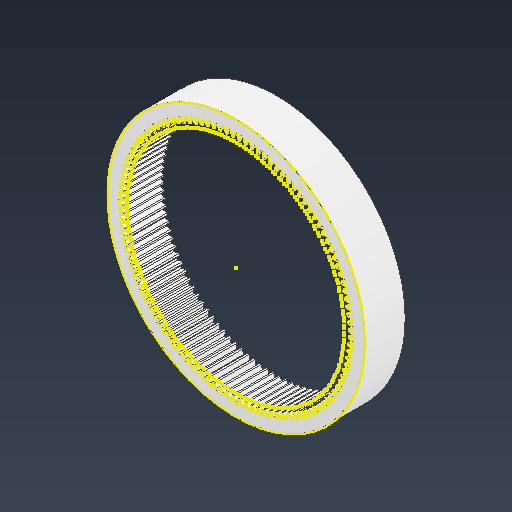
# Autodesk Inventor part: 平歯車2
Saved by Autodesk Inventor 2021 (Build 250183000, 183)
## iProperties
CustomPartVersion: 1
Created: 2021-08-20
Part Number: 平歯車2
Material: Steel
Document SubType Name: Modeling
Designer: yuta0
Categories: <?xml version="1.0" encoding="UTF-16"?> <MemberInstance><Categories><FamilyTemplate><FamilyTemplateParameter ValueType="xs:double" Id="1" ObjectReferenceKey="da_z" ObjectType="kUserParameterObject"/><FamilyTemplateParameter ValueType="xs:double" Id="2" ObjectReferenceKey="da_b" ObjectType="kUserParameterObject"/><FamilyTemplateParameter ValueType="xs:double" Id="3" ObjectReferenceKey="da_beta" ObjectType="kUserParameterObject"/><FamilyTemplateParameter ValueType="xs:double" Id="4" ObjectReferenceKey="da_da" ObjectType="kUserParameterObject"/><FamilyTemplateParameter ValueType="xs:double" Id="5" ObjectReferenceKey="da_aw" ObjectType="kUserParameterObject"/><FamilyTemplateParameter ValueType="xs:string" Id="6" ObjectReferenceKey="EAIAABAAAACIAQAAAAAAAIAAAAAAAAAA" ObjectType="83910656" SubObjectId="SurfaceGeometry"/></FamilyTemplate><ParamToTemplateMap><ParamToTemplate CategoryParameter="//CategoryParameter[@InternalName='046C89C9-8512-4d59-83FE-43B91F4F132A']" TemplateParameter="1"/><ParamToTemplate CategoryParameter="//CategoryParameter[@InternalName='2552DF32-E462-4b46-AEBF-C6C7768E72AC']" TemplateParameter="2"/><ParamToTemplate CategoryParameter="//CategoryParameter[@InternalName='C9EE641D-15FC-4fae-A226-E94C4372FDD7']" TemplateParameter="3"/><ParamToTemplate><ParamToTemplate CategoryParameter="//CategoryParameter[@InternalName='00B6519A-459B-49c7-AD84-2E56D39A5744']" ConstantValue="0.135415"/></ParamToTemplate><ParamToTemplate><ParamToTemplate CategoryParameter="//CategoryParameter[@InternalName='04B31F0E-C7A6-4894-AA32-9629BEFACF47']" ConstantValue="1.000000"/></ParamToTemplate><ParamToTemplate><ParamToTemplate CategoryParameter="//CategoryParameter[@InternalName='43CBEC2E-7847-49e7-A936-2F7889FCB2D9']" ConstantValue="0.250000"/></ParamToTemplate><ParamToTemplate><ParamToTemplate CategoryParameter="//CategoryParameter[@InternalName='B1EFC894-105D-4ebd-86BF-FA20ED196853']" ConstantValue="0.350000"/></ParamToTemplate><ParamToTemplate><ParamToTemplate CategoryParameter="//CategoryParameter[@InternalName='51175063-3D10-4879-93E8-6246FE8B403D']" ConstantValue="2060000000.000000"/></ParamToTemplate><ParamToTemplate><ParamToTemplate CategoryParameter="//CategoryParameter[@InternalName='A3A52E27-4454-46a9-B0BD-C932399B70AF']" ConstantValue="0.300000"/></ParamToTemplate><ParamToTemplate><ParamToTemplate CategoryParameter="//CategoryParameter[@InternalName='91B76062-C214-41d9-B1B9-14D2AB99603D']" ConstantValue="0.100000"/></ParamToTemplate><ParamToTemplate><ParamToTemplate CategoryParameter="//CategoryParameter[@InternalName='374E806E-8B8A-4dda-A9AA-1039D6500AD2']" ConstantValue="10.000000"/></ParamToTemplate><ParamToTemplate><ParamToTemplate CategoryParameter="//CategoryParameter[@InternalName='2D373A89-B862-43d6-8D0B-0CBF12AB9F6C']" ConstantValue="0.349066"/></ParamToTemplate><ParamToTemplate CategoryParameter="//CategoryParameter[@InternalName='37777632-D6A2-4fac-9D53-DB8ACD95C989']" TemplateParameter="4"/><ParamToTemplate CategoryParameter="//CategoryParameter[@InternalName='FD1017F1-B727-4f7e-9707-0F86F1FF9423']" TemplateParameter="5"/><ParamToTemplate><ParamToTemplate CategoryParameter="//CategoryParameter[@InternalName='9E1B4470-B2D3-4ff1-B813-535BB4CDF51A']" ConstantValue="3520000.000000"/></ParamToTemplate><ParamToTemplate><ParamToTemplate CategoryParameter="//CategoryParameter[@InternalName='F8452263-BFF6-458c-9FB1-07C4B99E95CD']" ConstantValue="11400000.000000"/></ParamToTemplate><ParamToTemplate><ParamToTemplate CategoryParameter="//CategoryParameter[@InternalName='3E3BB259-FD49-497f-8171-6EBC954A3479']" ConstantValue="2.000000"/></ParamToTemplate><ParamToTemplate CategoryParameter="//CategoryParameter[@InternalName='27C3BAF2-7550-4e4b-AE2C-0DB134B7D9B7']" TemplateParameter="6"/></ParamToTemplateMap><Category DisplayName="Gear" InternalName="DC85795E-93AB-48d5-8EEE-5A27447B64BD" Mnemonic="Gear"><CategoryParameter DisplayName="z" InternalName="046C89C9-8512-4d59-83FE-43B91F4F132A" Mnemonic="z"/><CategoryParameter DisplayName="b" InternalName="2552DF32-E462-4b46-AEBF-C6C7768E72AC" Mnemonic="b"/><CategoryParameter DisplayName="||b|" InternalName="C9EE641D-15FC-4fae-A226-E94C4372FDD7" Mnemonic="beta"/><CategoryParameter DisplayName="x" InternalName="00B6519A-459B-49c7-AD84-2E56D39A5744" Mnemonic="x"/><CategoryParameter DisplayName="a*" InternalName="04B31F0E-C7A6-4894-AA32-9629BEFACF47" Mnemonic="a"/><CategoryParameter DisplayName="c*" InternalName="43CBEC2E-7847-49e7-A936-2F7889FCB2D9" Mnemonic="c"/><CategoryParameter DisplayName="r|.f|*" InternalName="B1EFC894-105D-4ebd-86BF-FA20ED196853" Mnemonic="rf"/><CategoryParameter DisplayName="E" InternalName="51175063-3D10-4879-93E8-6246FE8B403D" Mnemonic="E"/><CategoryParameter DisplayName="||m|" InternalName="A3A52E27-4454-46a9-B0BD-C932399B70AF" Mnemonic="mi"/><Category DisplayName="SpurGear" InternalName="26C5A22E-A91E-4dfd-A3B3-23CCAFAE1764" Mnemonic="SpurGear"><CategoryParameter DisplayName="m" InternalName="91B76062-C214-41d9-B1B9-14D2AB99603D" Mnemonic="m"/><CategoryParameter DisplayName="P" InternalName="374E806E-8B8A-4dda-A9AA-1039D6500AD2" Mnemonic="PP"/><CategoryParameter DisplayName="||a|" InternalName="2D373A89-B862-43d6-8D0B-0CBF12AB9F6C" Mnemonic="alpha"/><CategoryParameter DisplayName="d|.a|" InternalName="37777632-D6A2-4fac-9D53-DB8ACD95C989" Mnemonic="da"/><CategoryParameter DisplayName="a|.w|" InternalName="FD1017F1-B727-4f7e-9707-0F86F1FF9423" Mnemonic="aw"/><CategoryParameter DisplayName="||s||.Flim|" InternalName="9E1B4470-B2D3-4ff1-B813-535BB4CDF51A" Mnemonic="sFlim"/><CategoryParameter DisplayName="||s||.Hlim|" InternalName="F8452263-BFF6-458c-9FB1-07C4B99E95CD" Mnemonic="sHlim"/><CategoryParameter DisplayName="種類" InternalName="3E3BB259-FD49-497f-8171-6EBC954A3479" Mnemonic="type"/><Category DisplayName="InternalSpurGear" InternalName="7CF704F6-14A9-42f8-93CE-E71DF57C2B55" Mnemonic="InternalSpurGear"><CategoryParameter DisplayName="PitchDiameter" InternalName="27C3BAF2-7550-4e4b-AE2C-0DB134B7D9B7" Mnemonic="IDS_PITCHDIAM"/></Category></Category></Category></Categories></MemberInstance>
Density: 1 g/cm^3
Appearance: 積雪
Author: yuta0
Autodesk Inventor part; units mm, degrees
sketch "Sketch1" plane through (0, 0, 0) normal (0, 0, 1) x (1, 0, 0)
  circle A0 centre (0, 0) radius 63.124
  dimension "d0" = 126.2479
  constraints: 1 centre point
  measures "d0" diameter of A0
extrude "Extrusion1" add sketch "Sketch1" along normal blind 20
ref_plane "Work Plane2" through (0, 0, 10) normal (0, 0, 1) x (1, 0, 0)
sketch "Sketch2" plane through (0, 0, 0) normal (0, 0, -1) x (-1, 0, 0)
  circle A0 centre (0, 0) radius 63.124 projected
  circle A1 centre (0, 0) radius 56
  dimension "d3" = 112
  constraints: 1 centre point, 1 coincident
  measures "d3" diameter of A1
surface extrude "ピッチ円直径" sketch "Sketch2" against normal through all shown no curves A1
ref_plane "Work Plane8" through (0, 0, 0) normal (0.9996066, 0.0280463, 0) x (0, 0, 1)
ref_plane "Work Plane9" through (0, 0, 0) normal (1, 0, 0) x (0, 1, 0)
spur gear teeth "平歯車" teeth 112 pitch diameter 112 tip diameter 110.2708 root diameter 114.7708 face width 20 start plane through (0, 0, 0) normal (0, 0, -1) x (-1, 0, 0)
sketch "スケッチ3" plane through (0, 0, 20) normal (0, 0, 1) x (1, 0, 0)
  arc A0 (3.6193, -57.2712) -> (4.2488, -54.9715) centre (-9.8202, -52.3566) ccw projected
  arc A1 (2.8158, -57.3163) -> (3.6193, -57.2712) centre (0, 0) ccw projected
  arc A2 (1.9328, -55.1015) -> (2.8158, -57.3163) centre (15.6206, -50.9279) ccw projected
  arc A3 (1.1598, -55.1232) -> (1.9328, -55.1015) centre (0, 0) ccw projected
  arc A4 (0.4024, -57.384) -> (1.1598, -55.1232) centre (-12.7405, -51.7236) ccw projected
  arc A5 (-0.4024, -57.384) -> (0.4024, -57.384) centre (0, 0) ccw projected
  arc A6 (-1.1598, -55.1232) -> (-0.4024, -57.384) centre (12.7405, -51.7236) ccw projected
  arc A7 (-1.9328, -55.1015) -> (-1.1598, -55.1232) centre (0, 0) ccw projected
  arc A8 (-2.8158, -57.3163) -> (-1.9328, -55.1015) centre (-15.6206, -50.9279) ccw projected
  arc A9 (-3.6193, -57.2712) -> (-2.8158, -57.3163) centre (0, 0) ccw projected
  arc A10 (-4.2488, -54.9715) -> (-3.6193, -57.2712) centre (9.8202, -52.3566) ccw projected
  arc A11 (-5.0193, -54.9065) -> (-4.2488, -54.9715) centre (0, 0) ccw projected
  arc A12 (-6.0251, -57.0682) -> (-5.0193, -54.9065) centre (-18.4516, -49.9719) ccw projected
  arc A13 (-6.8249, -56.9781) -> (-6.0251, -57.0682) centre (0, 0) ccw projected
  arc A14 (-7.3244, -54.6468) -> (-6.8249, -56.9781) centre (6.8691, -52.8248) ccw projected
  arc A15 (-8.09, -54.5387) -> (-7.3244, -54.6468) centre (0, 0) ccw projected
  arc A16 (-9.2155, -56.6406) -> (-8.09, -54.5387) centre (-21.2245, -48.8587) ccw projected
  arc A17 (-10.0089, -56.5058) -> (-9.2155, -56.6406) centre (0, 0) ccw projected
  arc A18 (-10.3769, -54.1501) -> (-10.0089, -56.5058) centre (3.8964, -53.1269) ccw projected
  arc A19 (-11.1353, -53.9992) -> (-10.3769, -54.1501) centre (0, 0) ccw projected
  arc A20 (-12.3768, -56.0348) -> (-11.1353, -53.9992) centre (-23.9306, -47.5918) ccw projected
  arc A21 (-13.1615, -55.8557) -> (-12.3768, -56.0348) centre (0, 0) ccw projected
  arc A22 (-13.3968, -53.4831) -> (-13.1615, -55.8557) centre (0.9114, -53.2618) ccw projected
  arc A23 (-14.1456, -53.2899) -> (-13.3968, -53.4831) centre (0, 0) ccw projected
  arc A24 (-15.4992, -55.2527) -> (-14.1456, -53.2899) centre (-26.5615, -46.1751) ccw projected
  arc A25 (-16.2726, -55.0299) -> (-15.4992, -55.2527) centre (0, 0) ccw projected
  arc A26 (-16.3746, -52.6478) -> (-16.2726, -55.0299) centre (-2.0764, -53.2291) ccw projected
  arc A27 (-17.1113, -52.4129) -> (-16.3746, -52.6478) centre (0, 0) ccw projected
  arc A28 (-18.5729, -54.2967) -> (-17.1113, -52.4129) centre (-29.1087, -44.6131) ccw projected
  arc A29 (-19.3326, -54.0309) -> (-18.5729, -54.2967) centre (0, 0) ccw projected
  arc A30 (-19.3008, -51.6468) -> (-19.3326, -54.0309) centre (-5.0577, -53.0289) ccw projected
  arc A31 (-20.0232, -51.3711) -> (-19.3008, -51.6468) centre (0, 0) ccw projected
  arc A32 (-21.5881, -53.1699) -> (-20.0232, -51.3711) centre (-31.5644, -42.9108) ccw projected
  arc A33 (-22.3317, -52.8619) -> (-21.5881, -53.1699) centre (0, 0) ccw projected
  arc A34 (-22.1663, -50.4834) -> (-22.3317, -52.8619) centre (-8.0231, -52.6619) ccw projected
  arc A35 (-22.8721, -50.1675) -> (-22.1663, -50.4834) centre (0, 0) ccw projected
  arc A36 (-24.5354, -51.8758) -> (-22.8721, -50.1675) centre (-33.9208, -41.0735) ccw projected
  arc A37 (-25.2605, -51.5266) -> (-24.5354, -51.8758) centre (0, 0) ccw projected
  arc A38 (-24.962, -49.1611) -> (-25.2605, -51.5266) centre (-10.9633, -52.1292) ccw projected
  arc A39 (-25.649, -48.8062) -> (-24.962, -49.1611) centre (0, 0) ccw projected
  arc A40 (-27.4055, -50.4185) -> (-25.649, -48.8062) centre (-36.1704, -39.1069) ccw projected
  arc A41 (-28.1099, -50.0292) -> (-27.4055, -50.4185) centre (0, 0) ccw projected
  arc A42 (-27.6792, -47.6841) -> (-28.1099, -50.0292) centre (-13.8689, -51.4325) ccw projected
  arc A43 (-28.3453, -47.2912) -> (-27.6792, -47.6841) centre (0, 0) ccw projected
  arc A44 (-30.1894, -48.8025) -> (-28.3453, -47.2912) centre (-38.3063, -37.0173) ccw projected
  arc A45 (-30.8709, -48.3743) -> (-30.1894, -48.8025) centre (0, 0) ccw projected
  arc A46 (-30.3094, -46.0571) -> (-30.8709, -48.3743) centre (-16.731, -50.574) ccw projected
  arc A47 (-30.9523, -45.6275) -> (-30.3094, -46.0571) centre (0, 0) ccw projected
  arc A48 (-32.8783, -47.033) -> (-30.9523, -45.6275) centre (-40.3216, -34.8112) ccw projected
  arc A49 (-33.5347, -46.5673) -> (-32.8783, -47.033) centre (0, 0) ccw projected
  arc A50 (-32.8441, -44.2852) -> (-33.5347, -46.5673) centre (-19.5403, -49.5563) ccw projected
  arc A51 (-33.462, -43.8202) -> (-32.8441, -44.2852) centre (0, 0) ccw projected
  arc A52 (-35.4637, -45.1155) -> (-33.462, -43.8202) centre (-42.21, -32.4956) ccw projected
  arc A53 (-36.093, -44.6137) -> (-35.4637, -45.1155) centre (0, 0) ccw projected
  arc A54 (-35.2755, -42.3739) -> (-36.093, -44.6137) centre (-22.2882, -48.3827) ccw projected
  arc A55 (-35.8664, -41.875) -> (-35.2755, -42.3739) centre (0, 0) ccw projected
  arc A56 (-37.9376, -43.0561) -> (-35.8664, -41.875) centre (-43.9657, -30.0777) ccw projected
  arc A57 (-38.5377, -42.5198) -> (-37.9376, -43.0561) centre (0, 0) ccw projected
  arc A58 (-37.596, -40.3293) -> (-38.5377, -42.5198) centre (-24.966, -47.0569) ccw projected
  arc A59 (-38.1579, -39.7981) -> (-37.596, -40.3293) centre (0, 0) ccw projected
  arc A60 (-40.2921, -40.8612) -> (-38.1579, -39.7981) centre (-45.583, -27.5652) ccw projected
  arc A61 (-40.8612, -40.2921) -> (-40.2921, -40.8612) centre (0, 0) ccw projected
  arc A62 (-39.7981, -38.1579) -> (-40.8612, -40.2921) centre (-27.5652, -45.583) ccw projected
  arc A63 (-40.3293, -37.596) -> (-39.7981, -38.1579) centre (0, 0) ccw projected
  arc A64 (-42.5198, -38.5377) -> (-40.3293, -37.596) centre (-47.0569, -24.966) ccw projected
  arc A65 (-43.0561, -37.9376) -> (-42.5198, -38.5377) centre (0, 0) ccw projected
  arc A66 (-41.875, -35.8664) -> (-43.0561, -37.9376) centre (-30.0777, -43.9657) ccw projected
  arc A67 (-42.3739, -35.2755) -> (-41.875, -35.8664) centre (0, 0) ccw projected
  arc A68 (-44.6137, -36.093) -> (-42.3739, -35.2755) centre (-48.3827, -22.2882) ccw projected
  arc A69 (-45.1155, -35.4637) -> (-44.6137, -36.093) centre (0, 0) ccw projected
  arc A70 (-43.8202, -33.462) -> (-45.1155, -35.4637) centre (-32.4956, -42.21) ccw projected
  arc A71 (-44.2852, -32.8441) -> (-43.8202, -33.462) centre (0, 0) ccw projected
  arc A72 (-46.5673, -33.5347) -> (-44.2852, -32.8441) centre (-49.5563, -19.5403) ccw projected
  arc A73 (-47.033, -32.8783) -> (-46.5673, -33.5347) centre (0, 0) ccw projected
  arc A74 (-45.6275, -30.9523) -> (-47.033, -32.8783) centre (-34.8112, -40.3216) ccw projected
  arc A75 (-46.0571, -30.3094) -> (-45.6275, -30.9523) centre (0, 0) ccw projected
  arc A76 (-48.3743, -30.8709) -> (-46.0571, -30.3094) centre (-50.574, -16.731) ccw projected
  arc A77 (-48.8025, -30.1894) -> (-48.3743, -30.8709) centre (0, 0) ccw projected
  arc A78 (-47.2912, -28.3453) -> (-48.8025, -30.1894) centre (-37.0173, -38.3063) ccw projected
  arc A79 (-47.6841, -27.6792) -> (-47.2912, -28.3453) centre (0, 0) ccw projected
  arc A80 (-50.0292, -28.1099) -> (-47.6841, -27.6792) centre (-51.4325, -13.8689) ccw projected
  arc A81 (-50.4185, -27.4055) -> (-50.0292, -28.1099) centre (0, 0) ccw projected
  arc A82 (-48.8062, -25.649) -> (-50.4185, -27.4055) centre (-39.1069, -36.1704) ccw projected
  arc A83 (-49.1611, -24.962) -> (-48.8062, -25.649) centre (0, 0) ccw projected
  arc A84 (-51.5266, -25.2605) -> (-49.1611, -24.962) centre (-52.1292, -10.9633) ccw projected
  arc A85 (-51.8758, -24.5354) -> (-51.5266, -25.2605) centre (0, 0) ccw projected
  arc A86 (-50.1675, -22.8721) -> (-51.8758, -24.5354) centre (-41.0735, -33.9208) ccw projected
  arc A87 (-50.4834, -22.1663) -> (-50.1675, -22.8721) centre (0, 0) ccw projected
  arc A88 (-52.8619, -22.3317) -> (-50.4834, -22.1663) centre (-52.6619, -8.0231) ccw projected
  arc A89 (-53.1699, -21.5881) -> (-52.8619, -22.3317) centre (0, 0) ccw projected
  arc A90 (-51.3711, -20.0232) -> (-53.1699, -21.5881) centre (-42.9108, -31.5644) ccw projected
  arc A91 (-51.6468, -19.3008) -> (-51.3711, -20.0232) centre (0, 0) ccw projected
  arc A92 (-54.0309, -19.3326) -> (-51.6468, -19.3008) centre (-53.0289, -5.0577) ccw projected
  arc A93 (-54.2967, -18.5729) -> (-54.0309, -19.3326) centre (0, 0) ccw projected
  arc A94 (-52.4129, -17.1113) -> (-54.2967, -18.5729) centre (-44.6131, -29.1087) ccw projected
  arc A95 (-52.6478, -16.3746) -> (-52.4129, -17.1113) centre (0, 0) ccw projected
  arc A96 (-55.0299, -16.2726) -> (-52.6478, -16.3746) centre (-53.2291, -2.0764) ccw projected
  arc A97 (-55.2527, -15.4992) -> (-55.0299, -16.2726) centre (0, 0) ccw projected
  arc A98 (-53.2899, -14.1456) -> (-55.2527, -15.4992) centre (-46.1751, -26.5615) ccw projected
  arc A99 (-53.4831, -13.3968) -> (-53.2899, -14.1456) centre (0, 0) ccw projected
  arc A100 (-55.8557, -13.1615) -> (-53.4831, -13.3968) centre (-53.2618, 0.9114) ccw projected
  arc A101 (-56.0348, -12.3768) -> (-55.8557, -13.1615) centre (0, 0) ccw projected
  arc A102 (-53.9992, -11.1353) -> (-56.0348, -12.3768) centre (-47.5918, -23.9306) ccw projected
  arc A103 (-54.1501, -10.3769) -> (-53.9992, -11.1353) centre (0, 0) ccw projected
  arc A104 (-56.5058, -10.0089) -> (-54.1501, -10.3769) centre (-53.1269, 3.8964) ccw projected
  arc A105 (-56.6406, -9.2155) -> (-56.5058, -10.0089) centre (0, 0) ccw projected
  arc A106 (-54.5387, -8.09) -> (-56.6406, -9.2155) centre (-48.8587, -21.2245) ccw projected
  arc A107 (-54.6468, -7.3244) -> (-54.5387, -8.09) centre (0, 0) ccw projected
  arc A108 (-56.9781, -6.8249) -> (-54.6468, -7.3244) centre (-52.8248, 6.8691) ccw projected
  arc A109 (-57.0682, -6.0251) -> (-56.9781, -6.8249) centre (0, 0) ccw projected
  arc A110 (-54.9065, -5.0193) -> (-57.0682, -6.0251) centre (-49.9719, -18.4516) ccw projected
  arc A111 (-54.9715, -4.2488) -> (-54.9065, -5.0193) centre (0, 0) ccw projected
  arc A112 (-57.2712, -3.6193) -> (-54.9715, -4.2488) centre (-52.3566, 9.8202) ccw projected
  arc A113 (-57.3163, -2.8158) -> (-57.2712, -3.6193) centre (0, 0) ccw projected
  arc A114 (-55.1015, -1.9328) -> (-57.3163, -2.8158) centre (-50.9279, -15.6206) ccw projected
  arc A115 (-55.1232, -1.1598) -> (-55.1015, -1.9328) centre (0, 0) ccw projected
  arc A116 (-57.384, -0.4024) -> (-55.1232, -1.1598) centre (-51.7236, 12.7405) ccw projected
  arc A117 (-57.384, 0.4024) -> (-57.384, -0.4024) centre (0, 0) ccw projected
  arc A118 (-55.1232, 1.1598) -> (-57.384, 0.4024) centre (-51.7236, -12.7405) ccw projected
  arc A119 (-55.1015, 1.9328) -> (-55.1232, 1.1598) centre (0, 0) ccw projected
  arc A120 (-57.3163, 2.8158) -> (-55.1015, 1.9328) centre (-50.9279, 15.6206) ccw projected
  arc A121 (-57.2712, 3.6193) -> (-57.3163, 2.8158) centre (0, 0) ccw projected
  arc A122 (-54.9715, 4.2488) -> (-57.2712, 3.6193) centre (-52.3566, -9.8202) ccw projected
  arc A123 (-54.9065, 5.0193) -> (-54.9715, 4.2488) centre (0, 0) ccw projected
  arc A124 (-57.0682, 6.0251) -> (-54.9065, 5.0193) centre (-49.9719, 18.4516) ccw projected
  arc A125 (-56.9781, 6.8249) -> (-57.0682, 6.0251) centre (0, 0) ccw projected
  arc A126 (-54.6468, 7.3244) -> (-56.9781, 6.8249) centre (-52.8248, -6.8691) ccw projected
  arc A127 (-54.5387, 8.09) -> (-54.6468, 7.3244) centre (0, 0) ccw projected
  arc A128 (-56.6406, 9.2155) -> (-54.5387, 8.09) centre (-48.8587, 21.2245) ccw projected
  arc A129 (-56.5058, 10.0089) -> (-56.6406, 9.2155) centre (0, 0) ccw projected
  arc A130 (-54.1501, 10.3769) -> (-56.5058, 10.0089) centre (-53.1269, -3.8964) ccw projected
  arc A131 (-53.9992, 11.1353) -> (-54.1501, 10.3769) centre (0, 0) ccw projected
  arc A132 (-56.0348, 12.3768) -> (-53.9992, 11.1353) centre (-47.5918, 23.9306) ccw projected
  arc A133 (-55.8557, 13.1615) -> (-56.0348, 12.3768) centre (0, 0) ccw projected
  arc A134 (-53.4831, 13.3968) -> (-55.8557, 13.1615) centre (-53.2618, -0.9114) ccw projected
  arc A135 (-53.2899, 14.1456) -> (-53.4831, 13.3968) centre (0, 0) ccw projected
  arc A136 (-55.2527, 15.4992) -> (-53.2899, 14.1456) centre (-46.1751, 26.5615) ccw projected
  arc A137 (-55.0299, 16.2726) -> (-55.2527, 15.4992) centre (0, 0) ccw projected
  arc A138 (-52.6478, 16.3746) -> (-55.0299, 16.2726) centre (-53.2291, 2.0764) ccw projected
  arc A139 (-52.4129, 17.1113) -> (-52.6478, 16.3746) centre (0, 0) ccw projected
  arc A140 (-54.2967, 18.5729) -> (-52.4129, 17.1113) centre (-44.6131, 29.1087) ccw projected
  arc A141 (-54.0309, 19.3326) -> (-54.2967, 18.5729) centre (0, 0) ccw projected
  arc A142 (-51.6468, 19.3008) -> (-54.0309, 19.3326) centre (-53.0289, 5.0577) ccw projected
  arc A143 (-51.3711, 20.0232) -> (-51.6468, 19.3008) centre (0, 0) ccw projected
  arc A144 (-53.1699, 21.5881) -> (-51.3711, 20.0232) centre (-42.9108, 31.5644) ccw projected
  arc A145 (-52.8619, 22.3317) -> (-53.1699, 21.5881) centre (0, 0) ccw projected
  arc A146 (-50.4834, 22.1663) -> (-52.8619, 22.3317) centre (-52.6619, 8.0231) ccw projected
  arc A147 (-50.1675, 22.8721) -> (-50.4834, 22.1663) centre (0, 0) ccw projected
  arc A148 (-51.8758, 24.5354) -> (-50.1675, 22.8721) centre (-41.0735, 33.9208) ccw projected
  arc A149 (-51.5266, 25.2605) -> (-51.8758, 24.5354) centre (0, 0) ccw projected
  arc A150 (-49.1611, 24.962) -> (-51.5266, 25.2605) centre (-52.1292, 10.9633) ccw projected
  arc A151 (-48.8062, 25.649) -> (-49.1611, 24.962) centre (0, 0) ccw projected
  arc A152 (-50.4185, 27.4055) -> (-48.8062, 25.649) centre (-39.1069, 36.1704) ccw projected
  arc A153 (-50.0292, 28.1099) -> (-50.4185, 27.4055) centre (0, 0) ccw projected
  arc A154 (-47.6841, 27.6792) -> (-50.0292, 28.1099) centre (-51.4325, 13.8689) ccw projected
  arc A155 (-47.2912, 28.3453) -> (-47.6841, 27.6792) centre (0, 0) ccw projected
  arc A156 (-48.8025, 30.1894) -> (-47.2912, 28.3453) centre (-37.0173, 38.3063) ccw projected
  arc A157 (-48.3743, 30.8709) -> (-48.8025, 30.1894) centre (0, 0) ccw projected
  arc A158 (-46.0571, 30.3094) -> (-48.3743, 30.8709) centre (-50.574, 16.731) ccw projected
  arc A159 (-45.6275, 30.9523) -> (-46.0571, 30.3094) centre (0, 0) ccw projected
  arc A160 (-47.033, 32.8783) -> (-45.6275, 30.9523) centre (-34.8112, 40.3216) ccw projected
  arc A161 (-46.5673, 33.5347) -> (-47.033, 32.8783) centre (0, 0) ccw projected
  arc A162 (-44.2852, 32.8441) -> (-46.5673, 33.5347) centre (-49.5563, 19.5403) ccw projected
  arc A163 (-43.8202, 33.462) -> (-44.2852, 32.8441) centre (0, 0) ccw projected
  arc A164 (-45.1155, 35.4637) -> (-43.8202, 33.462) centre (-32.4956, 42.21) ccw projected
  arc A165 (-44.6137, 36.093) -> (-45.1155, 35.4637) centre (0, 0) ccw projected
  arc A166 (-42.3739, 35.2755) -> (-44.6137, 36.093) centre (-48.3827, 22.2882) ccw projected
  arc A167 (-41.875, 35.8664) -> (-42.3739, 35.2755) centre (0, 0) ccw projected
  arc A168 (-43.0561, 37.9376) -> (-41.875, 35.8664) centre (-30.0777, 43.9657) ccw projected
  arc A169 (-42.5198, 38.5377) -> (-43.0561, 37.9376) centre (0, 0) ccw projected
  arc A170 (-40.3293, 37.596) -> (-42.5198, 38.5377) centre (-47.0569, 24.966) ccw projected
  arc A171 (-39.7981, 38.1579) -> (-40.3293, 37.596) centre (0, 0) ccw projected
  arc A172 (-40.8612, 40.2921) -> (-39.7981, 38.1579) centre (-27.5652, 45.583) ccw projected
  arc A173 (-40.2921, 40.8612) -> (-40.8612, 40.2921) centre (0, 0) ccw projected
  arc A174 (-38.1579, 39.7981) -> (-40.2921, 40.8612) centre (-45.583, 27.5652) ccw projected
  arc A175 (-37.596, 40.3293) -> (-38.1579, 39.7981) centre (0, 0) ccw projected
  arc A176 (-38.5377, 42.5198) -> (-37.596, 40.3293) centre (-24.966, 47.0569) ccw projected
  arc A177 (-37.9376, 43.0561) -> (-38.5377, 42.5198) centre (0, 0) ccw projected
  arc A178 (-35.8664, 41.875) -> (-37.9376, 43.0561) centre (-43.9657, 30.0777) ccw projected
  arc A179 (-35.2755, 42.3739) -> (-35.8664, 41.875) centre (0, 0) ccw projected
  arc A180 (-36.093, 44.6137) -> (-35.2755, 42.3739) centre (-22.2882, 48.3827) ccw projected
  arc A181 (-35.4637, 45.1155) -> (-36.093, 44.6137) centre (0, 0) ccw projected
  arc A182 (-33.462, 43.8202) -> (-35.4637, 45.1155) centre (-42.21, 32.4956) ccw projected
  arc A183 (-32.8441, 44.2852) -> (-33.462, 43.8202) centre (0, 0) ccw projected
  arc A184 (-33.5347, 46.5673) -> (-32.8441, 44.2852) centre (-19.5403, 49.5563) ccw projected
  arc A185 (-32.8783, 47.033) -> (-33.5347, 46.5673) centre (0, 0) ccw projected
  arc A186 (-30.9523, 45.6275) -> (-32.8783, 47.033) centre (-40.3216, 34.8112) ccw projected
  arc A187 (-30.3094, 46.0571) -> (-30.9523, 45.6275) centre (0, 0) ccw projected
  arc A188 (-30.8709, 48.3743) -> (-30.3094, 46.0571) centre (-16.731, 50.574) ccw projected
  arc A189 (-30.1894, 48.8025) -> (-30.8709, 48.3743) centre (0, 0) ccw projected
  arc A190 (-28.3453, 47.2912) -> (-30.1894, 48.8025) centre (-38.3063, 37.0173) ccw projected
  arc A191 (-27.6792, 47.6841) -> (-28.3453, 47.2912) centre (0, 0) ccw projected
  arc A192 (-28.1099, 50.0292) -> (-27.6792, 47.6841) centre (-13.8689, 51.4325) ccw projected
  arc A193 (-27.4055, 50.4185) -> (-28.1099, 50.0292) centre (0, 0) ccw projected
  arc A194 (-25.649, 48.8062) -> (-27.4055, 50.4185) centre (-36.1704, 39.1069) ccw projected
  arc A195 (-24.962, 49.1611) -> (-25.649, 48.8062) centre (0, 0) ccw projected
  arc A196 (-25.2605, 51.5266) -> (-24.962, 49.1611) centre (-10.9633, 52.1292) ccw projected
  arc A197 (-24.5354, 51.8758) -> (-25.2605, 51.5266) centre (0, 0) ccw projected
  arc A198 (-22.8721, 50.1675) -> (-24.5354, 51.8758) centre (-33.9208, 41.0735) ccw projected
  arc A199 (-22.1663, 50.4834) -> (-22.8721, 50.1675) centre (0, 0) ccw projected
  arc A200 (-22.3317, 52.8619) -> (-22.1663, 50.4834) centre (-8.0231, 52.6619) ccw projected
  arc A201 (-21.5881, 53.1699) -> (-22.3317, 52.8619) centre (0, 0) ccw projected
  arc A202 (-20.0232, 51.3711) -> (-21.5881, 53.1699) centre (-31.5644, 42.9108) ccw projected
  arc A203 (-19.3008, 51.6468) -> (-20.0232, 51.3711) centre (0, 0) ccw projected
  arc A204 (-19.3326, 54.0309) -> (-19.3008, 51.6468) centre (-5.0577, 53.0289) ccw projected
  arc A205 (-18.5729, 54.2967) -> (-19.3326, 54.0309) centre (0, 0) ccw projected
  arc A206 (-17.1113, 52.4129) -> (-18.5729, 54.2967) centre (-29.1087, 44.6131) ccw projected
  arc A207 (-16.3746, 52.6478) -> (-17.1113, 52.4129) centre (0, 0) ccw projected
  arc A208 (-16.2726, 55.0299) -> (-16.3746, 52.6478) centre (-2.0764, 53.2291) ccw projected
  arc A209 (-15.4992, 55.2527) -> (-16.2726, 55.0299) centre (0, 0) ccw projected
  arc A210 (-14.1456, 53.2899) -> (-15.4992, 55.2527) centre (-26.5615, 46.1751) ccw projected
  arc A211 (-13.3968, 53.4831) -> (-14.1456, 53.2899) centre (0, 0) ccw projected
  arc A212 (-13.1615, 55.8557) -> (-13.3968, 53.4831) centre (0.9114, 53.2618) ccw projected
  arc A213 (-12.3768, 56.0348) -> (-13.1615, 55.8557) centre (0, 0) ccw projected
  arc A214 (-11.1353, 53.9992) -> (-12.3768, 56.0348) centre (-23.9306, 47.5918) ccw projected
  arc A215 (-10.3769, 54.1501) -> (-11.1353, 53.9992) centre (0, 0) ccw projected
  arc A216 (-10.0089, 56.5058) -> (-10.3769, 54.1501) centre (3.8964, 53.1269) ccw projected
  arc A217 (-9.2155, 56.6406) -> (-10.0089, 56.5058) centre (0, 0) ccw projected
  arc A218 (-8.09, 54.5387) -> (-9.2155, 56.6406) centre (-21.2245, 48.8587) ccw projected
  arc A219 (-7.3244, 54.6468) -> (-8.09, 54.5387) centre (0, 0) ccw projected
  arc A220 (-6.8249, 56.9781) -> (-7.3244, 54.6468) centre (6.8691, 52.8248) ccw projected
  arc A221 (-6.0251, 57.0682) -> (-6.8249, 56.9781) centre (0, 0) ccw projected
  arc A222 (-5.0193, 54.9065) -> (-6.0251, 57.0682) centre (-18.4516, 49.9719) ccw projected
  arc A223 (-4.2488, 54.9715) -> (-5.0193, 54.9065) centre (0, 0) ccw projected
  arc A224 (-3.6193, 57.2712) -> (-4.2488, 54.9715) centre (9.8202, 52.3566) ccw projected
  arc A225 (-2.8158, 57.3163) -> (-3.6193, 57.2712) centre (0, 0) ccw projected
  arc A226 (-1.9328, 55.1015) -> (-2.8158, 57.3163) centre (-15.6206, 50.9279) ccw projected
  arc A227 (-1.1598, 55.1232) -> (-1.9328, 55.1015) centre (0, 0) ccw projected
  arc A228 (-0.4024, 57.384) -> (-1.1598, 55.1232) centre (12.7405, 51.7236) ccw projected
  arc A229 (0.4024, 57.384) -> (-0.4024, 57.384) centre (0, 0) ccw projected
  arc A230 (1.1598, 55.1232) -> (0.4024, 57.384) centre (-12.7405, 51.7236) ccw projected
  arc A231 (1.9328, 55.1015) -> (1.1598, 55.1232) centre (0, 0) ccw projected
  arc A232 (2.8158, 57.3163) -> (1.9328, 55.1015) centre (15.6206, 50.9279) ccw projected
  arc A233 (3.6193, 57.2712) -> (2.8158, 57.3163) centre (0, 0) ccw projected
  arc A234 (4.2488, 54.9715) -> (3.6193, 57.2712) centre (-9.8202, 52.3566) ccw projected
  arc A235 (5.0193, 54.9065) -> (4.2488, 54.9715) centre (0, 0) ccw projected
  arc A236 (6.0251, 57.0682) -> (5.0193, 54.9065) centre (18.4516, 49.9719) ccw projected
  arc A237 (6.8249, 56.9781) -> (6.0251, 57.0682) centre (0, 0) ccw projected
  arc A238 (7.3244, 54.6468) -> (6.8249, 56.9781) centre (-6.8691, 52.8248) ccw projected
  arc A239 (8.09, 54.5387) -> (7.3244, 54.6468) centre (0, 0) ccw projected
  arc A240 (9.2155, 56.6406) -> (8.09, 54.5387) centre (21.2245, 48.8587) ccw projected
  arc A241 (10.0089, 56.5058) -> (9.2155, 56.6406) centre (0, 0) ccw projected
  arc A242 (10.3769, 54.1501) -> (10.0089, 56.5058) centre (-3.8964, 53.1269) ccw projected
  arc A243 (11.1353, 53.9992) -> (10.3769, 54.1501) centre (0, 0) ccw projected
  arc A244 (12.3768, 56.0348) -> (11.1353, 53.9992) centre (23.9306, 47.5918) ccw projected
  arc A245 (13.1615, 55.8557) -> (12.3768, 56.0348) centre (0, 0) ccw projected
  arc A246 (13.3968, 53.4831) -> (13.1615, 55.8557) centre (-0.9114, 53.2618) ccw projected
  arc A247 (14.1456, 53.2899) -> (13.3968, 53.4831) centre (0, 0) ccw projected
  arc A248 (15.4992, 55.2527) -> (14.1456, 53.2899) centre (26.5615, 46.1751) ccw projected
  arc A249 (16.2726, 55.0299) -> (15.4992, 55.2527) centre (0, 0) ccw projected
  arc A250 (16.3746, 52.6478) -> (16.2726, 55.0299) centre (2.0764, 53.2291) ccw projected
  arc A251 (17.1113, 52.4129) -> (16.3746, 52.6478) centre (0, 0) ccw projected
  arc A252 (18.5729, 54.2967) -> (17.1113, 52.4129) centre (29.1087, 44.6131) ccw projected
  arc A253 (19.3326, 54.0309) -> (18.5729, 54.2967) centre (0, 0) ccw projected
  arc A254 (19.3008, 51.6468) -> (19.3326, 54.0309) centre (5.0577, 53.0289) ccw projected
  arc A255 (20.0232, 51.3711) -> (19.3008, 51.6468) centre (0, 0) ccw projected
  arc A256 (21.5881, 53.1699) -> (20.0232, 51.3711) centre (31.5644, 42.9108) ccw projected
  arc A257 (22.3317, 52.8619) -> (21.5881, 53.1699) centre (0, 0) ccw projected
  arc A258 (22.1663, 50.4834) -> (22.3317, 52.8619) centre (8.0231, 52.6619) ccw projected
  arc A259 (22.8721, 50.1675) -> (22.1663, 50.4834) centre (0, 0) ccw projected
  arc A260 (24.5354, 51.8758) -> (22.8721, 50.1675) centre (33.9208, 41.0735) ccw projected
  arc A261 (25.2605, 51.5266) -> (24.5354, 51.8758) centre (0, 0) ccw projected
  arc A262 (24.962, 49.1611) -> (25.2605, 51.5266) centre (10.9633, 52.1292) ccw projected
  arc A263 (25.649, 48.8062) -> (24.962, 49.1611) centre (0, 0) ccw projected
  arc A264 (27.4055, 50.4185) -> (25.649, 48.8062) centre (36.1704, 39.1069) ccw projected
  arc A265 (28.1099, 50.0292) -> (27.4055, 50.4185) centre (0, 0) ccw projected
  arc A266 (27.6792, 47.6841) -> (28.1099, 50.0292) centre (13.8689, 51.4325) ccw projected
  arc A267 (28.3453, 47.2912) -> (27.6792, 47.6841) centre (0, 0) ccw projected
  arc A268 (30.1894, 48.8025) -> (28.3453, 47.2912) centre (38.3063, 37.0173) ccw projected
  arc A269 (30.8709, 48.3743) -> (30.1894, 48.8025) centre (0, 0) ccw projected
  arc A270 (30.3094, 46.0571) -> (30.8709, 48.3743) centre (16.731, 50.574) ccw projected
  arc A271 (30.9523, 45.6275) -> (30.3094, 46.0571) centre (0, 0) ccw projected
  arc A272 (32.8783, 47.033) -> (30.9523, 45.6275) centre (40.3216, 34.8112) ccw projected
  arc A273 (33.5347, 46.5673) -> (32.8783, 47.033) centre (0, 0) ccw projected
  arc A274 (32.8441, 44.2852) -> (33.5347, 46.5673) centre (19.5403, 49.5563) ccw projected
  arc A275 (33.462, 43.8202) -> (32.8441, 44.2852) centre (0, 0) ccw projected
  arc A276 (35.4637, 45.1155) -> (33.462, 43.8202) centre (42.21, 32.4956) ccw projected
  arc A277 (36.093, 44.6137) -> (35.4637, 45.1155) centre (0, 0) ccw projected
  arc A278 (35.2755, 42.3739) -> (36.093, 44.6137) centre (22.2882, 48.3827) ccw projected
  arc A279 (35.8664, 41.875) -> (35.2755, 42.3739) centre (0, 0) ccw projected
  arc A280 (37.9376, 43.0561) -> (35.8664, 41.875) centre (43.9657, 30.0777) ccw projected
  arc A281 (38.5377, 42.5198) -> (37.9376, 43.0561) centre (0, 0) ccw projected
  arc A282 (37.596, 40.3293) -> (38.5377, 42.5198) centre (24.966, 47.0569) ccw projected
  arc A283 (38.1579, 39.7981) -> (37.596, 40.3293) centre (0, 0) ccw projected
  arc A284 (40.2921, 40.8612) -> (38.1579, 39.7981) centre (45.583, 27.5652) ccw projected
  arc A285 (40.8612, 40.2921) -> (40.2921, 40.8612) centre (0, 0) ccw projected
  arc A286 (39.7981, 38.1579) -> (40.8612, 40.2921) centre (27.5652, 45.583) ccw projected
  arc A287 (40.3293, 37.596) -> (39.7981, 38.1579) centre (0, 0) ccw projected
  arc A288 (42.5198, 38.5377) -> (40.3293, 37.596) centre (47.0569, 24.966) ccw projected
  arc A289 (43.0561, 37.9376) -> (42.5198, 38.5377) centre (0, 0) ccw projected
  arc A290 (41.875, 35.8664) -> (43.0561, 37.9376) centre (30.0777, 43.9657) ccw projected
  arc A291 (42.3739, 35.2755) -> (41.875, 35.8664) centre (0, 0) ccw projected
  arc A292 (44.6137, 36.093) -> (42.3739, 35.2755) centre (48.3827, 22.2882) ccw projected
  arc A293 (45.1155, 35.4637) -> (44.6137, 36.093) centre (0, 0) ccw projected
  arc A294 (43.8202, 33.462) -> (45.1155, 35.4637) centre (32.4956, 42.21) ccw projected
  arc A295 (44.2852, 32.8441) -> (43.8202, 33.462) centre (0, 0) ccw projected
  arc A296 (46.5673, 33.5347) -> (44.2852, 32.8441) centre (49.5563, 19.5403) ccw projected
  arc A297 (47.033, 32.8783) -> (46.5673, 33.5347) centre (0, 0) ccw projected
  arc A298 (45.6275, 30.9523) -> (47.033, 32.8783) centre (34.8112, 40.3216) ccw projected
  arc A299 (46.0571, 30.3094) -> (45.6275, 30.9523) centre (0, 0) ccw projected
  arc A300 (48.3743, 30.8709) -> (46.0571, 30.3094) centre (50.574, 16.731) ccw projected
  arc A301 (48.8025, 30.1894) -> (48.3743, 30.8709) centre (0, 0) ccw projected
  arc A302 (47.2912, 28.3453) -> (48.8025, 30.1894) centre (37.0173, 38.3063) ccw projected
  arc A303 (47.6841, 27.6792) -> (47.2912, 28.3453) centre (0, 0) ccw projected
  arc A304 (50.0292, 28.1099) -> (47.6841, 27.6792) centre (51.4325, 13.8689) ccw projected
  arc A305 (50.4185, 27.4055) -> (50.0292, 28.1099) centre (0, 0) ccw projected
  arc A306 (48.8062, 25.649) -> (50.4185, 27.4055) centre (39.1069, 36.1704) ccw projected
  arc A307 (49.1611, 24.962) -> (48.8062, 25.649) centre (0, 0) ccw projected
  arc A308 (51.5266, 25.2605) -> (49.1611, 24.962) centre (52.1292, 10.9633) ccw projected
  arc A309 (51.8758, 24.5354) -> (51.5266, 25.2605) centre (0, 0) ccw projected
  arc A310 (50.1675, 22.8721) -> (51.8758, 24.5354) centre (41.0735, 33.9208) ccw projected
  arc A311 (50.4834, 22.1663) -> (50.1675, 22.8721) centre (0, 0) ccw projected
  arc A312 (52.8619, 22.3317) -> (50.4834, 22.1663) centre (52.6619, 8.0231) ccw projected
  arc A313 (53.1699, 21.5881) -> (52.8619, 22.3317) centre (0, 0) ccw projected
  arc A314 (51.3711, 20.0232) -> (53.1699, 21.5881) centre (42.9108, 31.5644) ccw projected
  arc A315 (51.6468, 19.3008) -> (51.3711, 20.0232) centre (0, 0) ccw projected
  arc A316 (54.0309, 19.3326) -> (51.6468, 19.3008) centre (53.0289, 5.0577) ccw projected
  arc A317 (54.2967, 18.5729) -> (54.0309, 19.3326) centre (0, 0) ccw projected
  arc A318 (52.4129, 17.1113) -> (54.2967, 18.5729) centre (44.6131, 29.1087) ccw projected
  arc A319 (52.6478, 16.3746) -> (52.4129, 17.1113) centre (0, 0) ccw projected
  arc A320 (55.0299, 16.2726) -> (52.6478, 16.3746) centre (53.2291, 2.0764) ccw projected
  arc A321 (55.2527, 15.4992) -> (55.0299, 16.2726) centre (0, 0) ccw projected
  arc A322 (53.2899, 14.1456) -> (55.2527, 15.4992) centre (46.1751, 26.5615) ccw projected
  arc A323 (53.4831, 13.3968) -> (53.2899, 14.1456) centre (0, 0) ccw projected
  arc A324 (55.8557, 13.1615) -> (53.4831, 13.3968) centre (53.2618, -0.9114) ccw projected
  arc A325 (56.0348, 12.3768) -> (55.8557, 13.1615) centre (0, 0) ccw projected
  arc A326 (53.9992, 11.1353) -> (56.0348, 12.3768) centre (47.5918, 23.9306) ccw projected
  arc A327 (54.1501, 10.3769) -> (53.9992, 11.1353) centre (0, 0) ccw projected
  arc A328 (56.5058, 10.0089) -> (54.1501, 10.3769) centre (53.1269, -3.8964) ccw projected
  arc A329 (56.6406, 9.2155) -> (56.5058, 10.0089) centre (0, 0) ccw projected
  arc A330 (54.5387, 8.09) -> (56.6406, 9.2155) centre (48.8587, 21.2245) ccw projected
  arc A331 (54.6468, 7.3244) -> (54.5387, 8.09) centre (0, 0) ccw projected
  arc A332 (56.9781, 6.8249) -> (54.6468, 7.3244) centre (52.8248, -6.8691) ccw projected
  arc A333 (57.0682, 6.0251) -> (56.9781, 6.8249) centre (0, 0) ccw projected
  arc A334 (54.9065, 5.0193) -> (57.0682, 6.0251) centre (49.9719, 18.4516) ccw projected
  arc A335 (54.9715, 4.2488) -> (54.9065, 5.0193) centre (0, 0) ccw projected
  arc A336 (57.2712, 3.6193) -> (54.9715, 4.2488) centre (52.3566, -9.8202) ccw projected
  arc A337 (57.3163, 2.8158) -> (57.2712, 3.6193) centre (0, 0) ccw projected
  arc A338 (55.1015, 1.9328) -> (57.3163, 2.8158) centre (50.9279, 15.6206) ccw projected
  arc A339 (55.1232, 1.1598) -> (55.1015, 1.9328) centre (0, 0) ccw projected
  arc A340 (57.384, 0.4024) -> (55.1232, 1.1598) centre (51.7236, -12.7405) ccw projected
  arc A341 (57.384, -0.4024) -> (57.384, 0.4024) centre (0, 0) ccw projected
  arc A342 (55.1232, -1.1598) -> (57.384, -0.4024) centre (51.7236, 12.7405) ccw projected
  arc A343 (55.1015, -1.9328) -> (55.1232, -1.1598) centre (0, 0) ccw projected
  arc A344 (57.3163, -2.8158) -> (55.1015, -1.9328) centre (50.9279, -15.6206) ccw projected
  arc A345 (57.2712, -3.6193) -> (57.3163, -2.8158) centre (0, 0) ccw projected
  arc A346 (54.9715, -4.2488) -> (57.2712, -3.6193) centre (52.3566, 9.8202) ccw projected
  arc A347 (54.9065, -5.0193) -> (54.9715, -4.2488) centre (0, 0) ccw projected
  arc A348 (57.0682, -6.0251) -> (54.9065, -5.0193) centre (49.9719, -18.4516) ccw projected
  arc A349 (56.9781, -6.8249) -> (57.0682, -6.0251) centre (0, 0) ccw projected
  arc A350 (54.6468, -7.3244) -> (56.9781, -6.8249) centre (52.8248, 6.8691) ccw projected
  arc A351 (54.5387, -8.09) -> (54.6468, -7.3244) centre (0, 0) ccw projected
  arc A352 (56.6406, -9.2155) -> (54.5387, -8.09) centre (48.8587, -21.2245) ccw projected
  arc A353 (56.5058, -10.0089) -> (56.6406, -9.2155) centre (0, 0) ccw projected
  arc A354 (54.1501, -10.3769) -> (56.5058, -10.0089) centre (53.1269, 3.8964) ccw projected
  arc A355 (53.9992, -11.1353) -> (54.1501, -10.3769) centre (0, 0) ccw projected
  arc A356 (56.0348, -12.3768) -> (53.9992, -11.1353) centre (47.5918, -23.9306) ccw projected
  arc A357 (55.8557, -13.1615) -> (56.0348, -12.3768) centre (0, 0) ccw projected
  arc A358 (53.4831, -13.3968) -> (55.8557, -13.1615) centre (53.2618, 0.9114) ccw projected
  arc A359 (53.2899, -14.1456) -> (53.4831, -13.3968) centre (0, 0) ccw projected
  arc A360 (55.2527, -15.4992) -> (53.2899, -14.1456) centre (46.1751, -26.5615) ccw projected
  arc A361 (55.0299, -16.2726) -> (55.2527, -15.4992) centre (0, 0) ccw projected
  arc A362 (52.6478, -16.3746) -> (55.0299, -16.2726) centre (53.2291, -2.0764) ccw projected
  arc A363 (52.4129, -17.1113) -> (52.6478, -16.3746) centre (0, 0) ccw projected
  arc A364 (54.2967, -18.5729) -> (52.4129, -17.1113) centre (44.6131, -29.1087) ccw projected
  arc A365 (54.0309, -19.3326) -> (54.2967, -18.5729) centre (0, 0) ccw projected
  arc A366 (51.6468, -19.3008) -> (54.0309, -19.3326) centre (53.0289, -5.0577) ccw projected
  arc A367 (51.3711, -20.0232) -> (51.6468, -19.3008) centre (0, 0) ccw projected
  arc A368 (53.1699, -21.5881) -> (51.3711, -20.0232) centre (42.9108, -31.5644) ccw projected
  arc A369 (52.8619, -22.3317) -> (53.1699, -21.5881) centre (0, 0) ccw projected
  arc A370 (50.4834, -22.1663) -> (52.8619, -22.3317) centre (52.6619, -8.0231) ccw projected
  arc A371 (50.1675, -22.8721) -> (50.4834, -22.1663) centre (0, 0) ccw projected
  arc A372 (51.8758, -24.5354) -> (50.1675, -22.8721) centre (41.0735, -33.9208) ccw projected
  arc A373 (51.5266, -25.2605) -> (51.8758, -24.5354) centre (0, 0) ccw projected
  arc A374 (49.1611, -24.962) -> (51.5266, -25.2605) centre (52.1292, -10.9633) ccw projected
  arc A375 (48.8062, -25.649) -> (49.1611, -24.962) centre (0, 0) ccw projected
  arc A376 (50.4185, -27.4055) -> (48.8062, -25.649) centre (39.1069, -36.1704) ccw projected
  arc A377 (50.0292, -28.1099) -> (50.4185, -27.4055) centre (0, 0) ccw projected
  arc A378 (47.6841, -27.6792) -> (50.0292, -28.1099) centre (51.4325, -13.8689) ccw projected
  arc A379 (47.2912, -28.3453) -> (47.6841, -27.6792) centre (0, 0) ccw projected
  arc A380 (48.8025, -30.1894) -> (47.2912, -28.3453) centre (37.0173, -38.3063) ccw projected
  arc A381 (48.3743, -30.8709) -> (48.8025, -30.1894) centre (0, 0) ccw projected
  arc A382 (46.0571, -30.3094) -> (48.3743, -30.8709) centre (50.574, -16.731) ccw projected
  arc A383 (45.6275, -30.9523) -> (46.0571, -30.3094) centre (0, 0) ccw projected
  arc A384 (47.033, -32.8783) -> (45.6275, -30.9523) centre (34.8112, -40.3216) ccw projected
  arc A385 (46.5673, -33.5347) -> (47.033, -32.8783) centre (0, 0) ccw projected
  arc A386 (44.2852, -32.8441) -> (46.5673, -33.5347) centre (49.5563, -19.5403) ccw projected
  arc A387 (43.8202, -33.462) -> (44.2852, -32.8441) centre (0, 0) ccw projected
  arc A388 (45.1155, -35.4637) -> (43.8202, -33.462) centre (32.4956, -42.21) ccw projected
  arc A389 (44.6137, -36.093) -> (45.1155, -35.4637) centre (0, 0) ccw projected
  arc A390 (42.3739, -35.2755) -> (44.6137, -36.093) centre (48.3827, -22.2882) ccw projected
  arc A391 (41.875, -35.8664) -> (42.3739, -35.2755) centre (0, 0) ccw projected
  arc A392 (43.0561, -37.9376) -> (41.875, -35.8664) centre (30.0777, -43.9657) ccw projected
  arc A393 (42.5198, -38.5377) -> (43.0561, -37.9376) centre (0, 0) ccw projected
  arc A394 (40.3293, -37.596) -> (42.5198, -38.5377) centre (47.0569, -24.966) ccw projected
  arc A395 (39.7981, -38.1579) -> (40.3293, -37.596) centre (0, 0) ccw projected
  arc A396 (40.8612, -40.2921) -> (39.7981, -38.1579) centre (27.5652, -45.583) ccw projected
  arc A397 (40.2921, -40.8612) -> (40.8612, -40.2921) centre (0, 0) ccw projected
  arc A398 (38.1579, -39.7981) -> (40.2921, -40.8612) centre (45.583, -27.5652) ccw projected
  arc A399 (37.596, -40.3293) -> (38.1579, -39.7981) centre (0, 0) ccw projected
  arc A400 (38.5377, -42.5198) -> (37.596, -40.3293) centre (24.966, -47.0569) ccw projected
  arc A401 (37.9376, -43.0561) -> (38.5377, -42.5198) centre (0, 0) ccw projected
  arc A402 (35.8664, -41.875) -> (37.9376, -43.0561) centre (43.9657, -30.0777) ccw projected
  arc A403 (35.2755, -42.3739) -> (35.8664, -41.875) centre (0, 0) ccw projected
  arc A404 (36.093, -44.6137) -> (35.2755, -42.3739) centre (22.2882, -48.3827) ccw projected
  arc A405 (35.4637, -45.1155) -> (36.093, -44.6137) centre (0, 0) ccw projected
  arc A406 (33.462, -43.8202) -> (35.4637, -45.1155) centre (42.21, -32.4956) ccw projected
  arc A407 (32.8441, -44.2852) -> (33.462, -43.8202) centre (0, 0) ccw projected
  arc A408 (33.5347, -46.5673) -> (32.8441, -44.2852) centre (19.5403, -49.5563) ccw projected
  arc A409 (32.8783, -47.033) -> (33.5347, -46.5673) centre (0, 0) ccw projected
  arc A410 (30.9523, -45.6275) -> (32.8783, -47.033) centre (40.3216, -34.8112) ccw projected
  arc A411 (30.3094, -46.0571) -> (30.9523, -45.6275) centre (0, 0) ccw projected
  arc A412 (30.8709, -48.3743) -> (30.3094, -46.0571) centre (16.731, -50.574) ccw projected
  arc A413 (30.1894, -48.8025) -> (30.8709, -48.3743) centre (0, 0) ccw projected
  arc A414 (28.3453, -47.2912) -> (30.1894, -48.8025) centre (38.3063, -37.0173) ccw projected
  arc A415 (27.6792, -47.6841) -> (28.3453, -47.2912) centre (0, 0) ccw projected
  arc A416 (28.1099, -50.0292) -> (27.6792, -47.6841) centre (13.8689, -51.4325) ccw projected
  arc A417 (27.4055, -50.4185) -> (28.1099, -50.0292) centre (0, 0) ccw projected
  arc A418 (25.649, -48.8062) -> (27.4055, -50.4185) centre (36.1704, -39.1069) ccw projected
  arc A419 (24.962, -49.1611) -> (25.649, -48.8062) centre (0, 0) ccw projected
  arc A420 (25.2605, -51.5266) -> (24.962, -49.1611) centre (10.9633, -52.1292) ccw projected
  arc A421 (24.5354, -51.8758) -> (25.2605, -51.5266) centre (0, 0) ccw projected
  arc A422 (22.8721, -50.1675) -> (24.5354, -51.8758) centre (33.9208, -41.0735) ccw projected
  arc A423 (22.1663, -50.4834) -> (22.8721, -50.1675) centre (0, 0) ccw projected
  arc A424 (22.3317, -52.8619) -> (22.1663, -50.4834) centre (8.0231, -52.6619) ccw projected
  arc A425 (21.5881, -53.1699) -> (22.3317, -52.8619) centre (0, 0) ccw projected
  arc A426 (20.0232, -51.3711) -> (21.5881, -53.1699) centre (31.5644, -42.9108) ccw projected
  arc A427 (19.3008, -51.6468) -> (20.0232, -51.3711) centre (0, 0) ccw projected
  arc A428 (19.3326, -54.0309) -> (19.3008, -51.6468) centre (5.0577, -53.0289) ccw projected
  arc A429 (18.5729, -54.2967) -> (19.3326, -54.0309) centre (0, 0) ccw projected
  arc A430 (17.1113, -52.4129) -> (18.5729, -54.2967) centre (29.1087, -44.6131) ccw projected
  arc A431 (16.3746, -52.6478) -> (17.1113, -52.4129) centre (0, 0) ccw projected
  arc A432 (16.2726, -55.0299) -> (16.3746, -52.6478) centre (2.0764, -53.2291) ccw projected
  arc A433 (15.4992, -55.2527) -> (16.2726, -55.0299) centre (0, 0) ccw projected
  arc A434 (14.1456, -53.2899) -> (15.4992, -55.2527) centre (26.5615, -46.1751) ccw projected
  arc A435 (13.3968, -53.4831) -> (14.1456, -53.2899) centre (0, 0) ccw projected
  arc A436 (13.1615, -55.8557) -> (13.3968, -53.4831) centre (-0.9114, -53.2618) ccw projected
  arc A437 (12.3768, -56.0348) -> (13.1615, -55.8557) centre (0, 0) ccw projected
  arc A438 (11.1353, -53.9992) -> (12.3768, -56.0348) centre (23.9306, -47.5918) ccw projected
  arc A439 (10.3769, -54.1501) -> (11.1353, -53.9992) centre (0, 0) ccw projected
  arc A440 (10.0089, -56.5058) -> (10.3769, -54.1501) centre (-3.8964, -53.1269) ccw projected
  arc A441 (9.2155, -56.6406) -> (10.0089, -56.5058) centre (0, 0) ccw projected
  arc A442 (8.09, -54.5387) -> (9.2155, -56.6406) centre (21.2245, -48.8587) ccw projected
  arc A443 (7.3244, -54.6468) -> (8.09, -54.5387) centre (0, 0) ccw projected
  arc A444 (6.8249, -56.9781) -> (7.3244, -54.6468) centre (-6.8691, -52.8248) ccw projected
  arc A445 (6.0251, -57.0682) -> (6.8249, -56.9781) centre (0, 0) ccw projected
  arc A446 (5.0193, -54.9065) -> (6.0251, -57.0682) centre (18.4516, -49.9719) ccw projected
  arc A447 (4.2488, -54.9715) -> (5.0193, -54.9065) centre (0, 0) ccw projected
  circle A448 centre (0, 0) radius 63.124 projected
equation "\"d0\" = 1.1 * da_df"
equation "\"d1\" = da_b"
equation "\"d3\" = da_d"
equation "\"d16\" = da_aw"
equation "\"d47\" = da_aw"
equation "\"d52\" = da_aw"
equation "\"da_df\" = 114.770829"
equation "\"da_b\" = 20"
equation "\"da_d\" = 112"
equation "\"da_aw\" = 32.133347"
body "Solid1"
body "Srf1"
